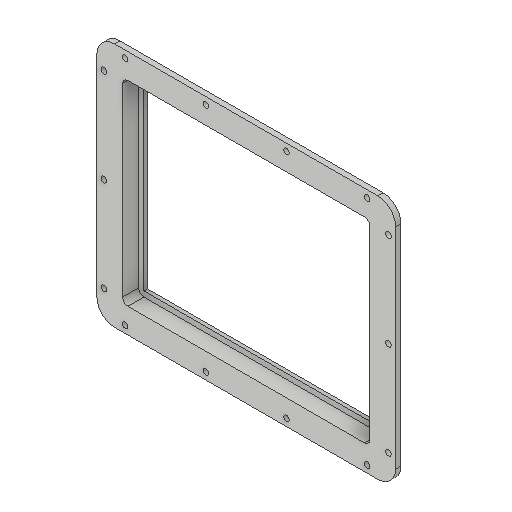
# Autodesk Inventor part: 3DP_PLA_Front_filter_mount_hood
Saved by Autodesk Inventor 2025 (Build 290162010, 162A)
## iProperties
Created: 2020-03-28
Part Number: 3DP_PLA_Front_filter_mount_hood
Material: Generic
Document SubType Name: Modeling
Designer: Andrzej
Density: 1 g/cm^3
Appearance: Default
Author: Andrzej
Autodesk Inventor part; units mm, degrees
ref_plane "YZ Plane" through (0, 0, 0) normal (1, 0, 0) x (0, 1, 0)
ref_plane "XZ Plane" through (0, 0, 0) normal (0, 1, 0) x (-1, 0, 0)
ref_plane "XY Plane" through (0, 0, 0) normal (0, 0, 1) x (1, 0, 0)
sketch "Sketch1" plane through (0, 0, 0) normal (0, 0, 1) x (1, 0, 0)
  line L0 (-76, 61) -> (76, 61)
  line L1 (76, 61) -> (76, -61)
  line L2 (76, -61) -> (-76, -61)
  line L3 (-76, -61) -> (-76, 61)
  line L4 (-69.5, 55) -> (69.5, 55)
  line L5 (69.5, 55) -> (69.5, -55)
  line L6 (69.5, -55) -> (-69.5, -55)
  line L7 (-69.5, -55) -> (-69.5, 55)
  line L8 (84, 69) -> (-84, 69)
  line L9 (-84, 69) -> (-84, -69)
  line L10 (-84, -69) -> (84, -69)
  line L11 (84, -69) -> (84, 69)
  line L12 (72.5, 58) -> (-72.5, 58)
  line L13 (-72.5, 58) -> (-72.5, -58)
  line L14 (-72.5, -58) -> (72.5, -58)
  line L15 (72.5, -58) -> (72.5, 58)
  line L16 (0, 109.6961) -> (0, -131.8013)
  line L17 (-145.0248, 0) -> (154.2595, 0)
  point P0 (0, 0)
  point P1 (-68, -65)
  point P2 (-80, -53)
  point P3 (-22.6667, -65)
  point P4 (22.6667, -65)
  point P5 (68, -65)
  point P6 (-80, 0)
  point P7 (-80, 53)
  point P8 (80, -53)
  point P9 (80, 0)
  point P10 (80, 53)
  point P11 (-68, 65)
  point P12 (-22.6667, 65)
  point P13 (22.6667, 65)
  point P14 (68, 65)
  dimension "d0" = 152
  dimension "d1" = 122
  dimension "d2" = 139
  dimension "d3" = 110
  dimension "d4" = 6
  dimension "d5" = 6.5
  dimension "d6" = 8
  dimension "d7" = 3
  dimension "d44" = 69.5
  dimension "d45" = 55
  dimension "d84" = 4
  dimension "d85" = 4
  dimension "d87" = 16
  dimension "d88" = 16
  dimension "d89" = 168
  dimension "d90" = 138
  dimension "d93" = 45.3333
  dimension "d100" = 53
  constraints: 36 end point, 8 parallel, 7 symmetric about line, 4 horizontal, 4 perpendicular, 2 vertical, 11 other
  measures "d0" distance of L1.end L2.end
  measures "d1" distance of L0.end L1.end
  measures "d2" distance of L5.end L6.end
  measures "d3" distance of L4.end L5.end
  measures "d4" distance between parallel lines of L0 L4
  measures "d5" distance between parallel lines of L3 L7
  measures "d6" distance between parallel lines of L0 L8
  measures "d7" distance between parallel lines of L4 L12
  measures "d44" distance from line of point (0, 0) L5
  measures "d45" distance from line of point (0, 0) L6
  measures "d84" distance from line of L2 point (-68, -65)
  measures "d85" distance from line of L3 point (-80, -53)
  measures "d87" distance from line of L9 point (-68, -65)
  measures "d88" distance from line of point (-80, -53) L10
  measures "d89" distance between parallel lines of L11 L9
  measures "d90" distance of L8.end L9.end
  measures "d93" distance of point (-68, -65) point (-22.667, -65)
  measures "d100" distance of point (-80, -53) point (-80, 0)
extrude "Extrusion1" add sketch "Sketch1" along normal blind 3 contours L3 L17 L9 L8 L16 L0 | L0 L16 L12 L13 L17 L3 | L16 L8 L11 L17 L1 L0 | L0 L1 L17 L15 L12 L16 | L17 L13 L14 L16 L2 L3 | L3 L2 L16 L10 L9 L17 | L16 L4 L7 L17 L13 L12 | L12 L15 L17 L5 L4 L16 | L17 L7 L6 L16 L14 L13 | L17 L11 L10 L16 L2 L1 | L1 L2 L16 L14 L15 L17 | L15 L14 L16 L6 L5 L17
extrude "Extrusion2" add sketch "Sketch1" against normal blind 8 contours L16 L4 L7 L17 L13 L12 | L12 L15 L17 L5 L4 L16 | L17 L7 L6 L16 L14 L13 | L15 L14 L16 L6 L5 L17
fillet "Fillet5" radius 3 8 edges at (72.5, 58, -4) (69.5, 55, -2.5) (-72.5, 58, -4) (-69.5, 55, -2.5) (-69.5, -55, -2.5) (-72.5, -58, -4) (72.5, -58, -4) (69.5, -55, -2.5)
fillet "Fillet6" radius 8 8 edges at (71.6213, 57.1213, 0) (0, 58, 0) (-71.6213, 57.1213, 0) (-72.5, 0, 0) (-71.6213, -57.1213, 0) (0, -58, 0) (71.6213, -57.1213, 0) (72.5, 0, 0)
fillet "Fillet8" radius 10 4 edges at (-84, -69, 1.5) (84, -69, 1.5) (84, 69, 1.5) (-84, 69, 1.5)
hole "Hole2" at (-68, -65, 0) at (-80, -53, 0) at (-22.6667, -65, 0) at (22.6667, -65, 0) at (68, -65, 0) at (-80, 0, 0) at (-80, 53, 0) at (80, 53, 0) at (80, 0, 0) at (80, -53, 0) at (-68, 65, 0) at (-22.6667, 65, 0) at (22.6667, 65, 0) at (68, 65, 0) direction (0, 0, 1) diameter 3.2 depth 3 tip angle 118
hole "Hole3" at (68, 65, 0) at (22.6667, 65, 0) at (-22.6667, 65, 0) at (-68, 65, 0) at (-80, 53, 0) at (-80, 0, 0) at (-80, -53, 0) at (-68, -65, 0) at (-22.6667, -65, 0) at (22.6667, -65, 0) at (68, -65, 0) at (80, -53, 0) at (80, 0, 0) at (80, 53, 0) direction (0, 0, -1) diameter 8 depth 5 tip angle 118
sketch "Sketch5" plane through (0, 0, -8) normal (0, 0, -1) x (-1, 0, 0)
  line L0 (69.5, 52) -> (69.5, -52) projected
  arc A0 (66.5, -55) -> (69.5, -52) centre (66.5, -52) ccw projected
  line L1 (66.5, -55) -> (-66.5, -55) projected
  arc A1 (-69.5, -52) -> (-66.5, -55) centre (-66.5, -52) ccw projected
  line L2 (-69.5, -52) -> (-69.5, 52) projected
  arc A2 (-66.5, 55) -> (-69.5, 52) centre (-66.5, 52) ccw projected
  line L3 (-66.5, 55) -> (66.5, 55) projected
  arc A3 (69.5, 52) -> (66.5, 55) centre (66.5, 52) ccw projected
  arc A4 (-72.5, -55) -> (-69.5, -58) centre (-69.5, -55) ccw projected
  line L4 (-69.5, -58) -> (69.5, -58) projected
  arc A5 (69.5, -58) -> (72.5, -55) centre (69.5, -55) ccw projected
  line L5 (72.5, -55) -> (72.5, 55) projected
  arc A6 (72.5, 55) -> (69.5, 58) centre (69.5, 55) ccw projected
  line L6 (69.5, 58) -> (-69.5, 58) projected
  arc A7 (-69.5, 58) -> (-72.5, 55) centre (-69.5, 55) ccw projected
  line L7 (-72.5, 55) -> (-72.5, -55) projected
  line L8 (-66.5, 52) -> (-66.5, -52)
  line L9 (-66.5, -52) -> (66.5, -52)
  line L10 (66.5, -52) -> (66.5, 52)
  line L11 (66.5, 52) -> (-66.5, 52)
  point P0 (0, 0)
  dimension "d119" = 3
  constraints: 8 end point, 3 other
  measures "d119" distance between parallel lines of L2 L8
extrude "Extrusion6" add sketch "Sketch5" against normal blind 2 contours L0 A0 L1 A1 L2 A2 L3 A3
equation "\"d4\" = -0.5 * d3 + 0.5 * d1"
equation "\"d5\" = -0.5 * d2 + 0.5 * d0"
equation "\"d44\" = 0.5 * d2"
equation "\"d45\" = 0.5 * d3"
equation "\"d84\" = 0.5 * d6"
equation "\"d85\" = d84"
equation "\"d88\" = d87"
equation "\"d93\" = -0.666667 * d87 + 0.333333 * d89"
equation "\"d100\" = -d88 + 0.5 * d90"
body "Solid1"
